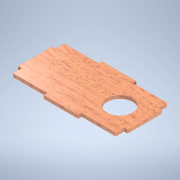
# Autodesk Inventor part: SideMale_120wx60h_V1
Saved by Autodesk Inventor 2022.2 (Build 262287000, 287)
## iProperties
Created: 2023-04-17
Part Number: SideMale_120wx60h_V1
Material: Wood (Oak)
Document SubType Name: Modeling
Designer: jaege
Density: 0.76 g/cm^3
Appearance: Red Oak - Natural Low Gloss
Author: jaege
Autodesk Inventor part; units mm, degrees
ref_plane "YZ Plane" through (0, 0, 0) normal (1, 0, 0) x (0, 1, 0)
ref_plane "XZ Plane" through (0, 0, 0) normal (0, 1, 0) x (-1, 0, 0)
ref_plane "XY Plane" through (0, 0, 0) normal (0, 0, 1) x (1, 0, 0)
sketch "Sketch1" plane through (0, 0, 0) normal (0, 1, 0) x (-1, 0, 0)
  line L0 (60, 30) -> (-60, 30) construction
  line L1 (-60, 30) -> (-60, -30) construction
  line L2 (-60, -30) -> (60, -30) construction
  line L3 (60, -30) -> (60, 30) construction
  line L4 (20, 30) -> (-20, 30) construction
  line L5 (-20, 30) -> (-20, 34)
  line L6 (-20, 34) -> (20, 34)
  line L7 (20, 34) -> (20, 30)
  line L8 (20, -30) -> (-20, -30) construction
  line L9 (-20, -30) -> (-20, -34)
  line L10 (-20, -34) -> (20, -34)
  line L11 (20, -34) -> (20, -30)
  line L12 (-60, -20) -> (-64, -20)
  line L13 (-64, -20) -> (-64, 20)
  line L14 (-64, 20) -> (-60, 20)
  line L15 (-60, 20) -> (-60, -20) construction
  line L16 (60, -20) -> (64, -20)
  line L17 (64, -20) -> (64, 20)
  line L18 (64, 20) -> (60, 20)
  line L19 (60, 20) -> (60, -20) construction
  line L20 (60, -20) -> (60, -30)
  line L21 (60, -30) -> (20, -30)
  line L22 (-20, -30) -> (-60, -30)
  line L23 (-60, -20) -> (-60, -30)
  line L24 (-60, 20) -> (-60, 30)
  line L25 (-20, 30) -> (-60, 30)
  line L26 (60, 20) -> (60, 30)
  line L27 (60, 30) -> (20, 30)
  point P0 (0, 0)
  point P1 (62, -20)
  point P2 (-62, 20)
  point P3 (62, 20)
  point P4 (0, -30)
  point P5 (0, 30)
  point P6 (60, 0)
  point P7 (-60, 0)
  point P8 (0, -30)
  point P9 (60, 0)
  dimension "d0" = 40
  dimension "d1" = 4
  dimension "d2" = 120
  dimension "d3" = 60
  constraints: 56 end point, 10 parallel, 9 collinear, 9 midpoint, 8 perpendicular, 5 horizontal, 5 horizontal alignment, 5 vertical alignment, 4 equal length
  measures "d0" distance of L9.end L10.end
  measures "d1" distance of L10.end L8.start
  measures "d2" distance between parallel lines of L1 L3
  measures "d3" distance of L0.end L1.end
extrude "Extrusion1" add sketch "Sketch1" along normal blind 4
sketch "Sketch2" plane through (0, 4, 0) normal (0, 1, 0) x (1, 0, 0)
  circle A0 centre (35, 0) radius 15
  line L0 (60, 20) -> (60, 30) projected
  point P0 (0, 0)
  dimension "d6" = 30
  dimension "d7" = 10
  constraints: 1 centre point, 1 horizontal alignment
  measures "d6" diameter of A0
  measures "d7" distance edge to line of A0 L0
extrude "Extrusion2" cut sketch "Sketch2" against normal blind 4
body "Solid1"
